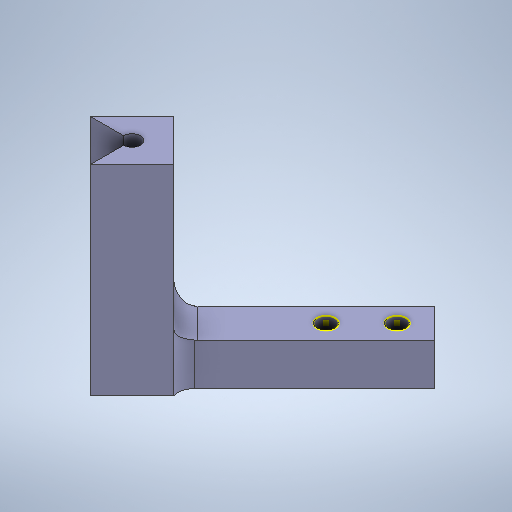
# Autodesk Inventor part: ALUMFINGER
Saved by Autodesk Inventor 2025.2 (Build 292293000, 293)
## iProperties
Created: 2025-02-25
Part Number: ALUMFINGER
Material: Generic
Document SubType Name: Modeling
Designer: m_kni
Density: 1 g/cm^3
Appearance: Default
Author: m_kni
## iProperties of the stored document ALUMFINGER_3DPrint.ipt
Created: 2025-03-03
Part Number: ALUMFINGER_3DPrint
Material: Generic
Document SubType Name: Modeling
Designer: m_kni
Density: 1 g/cm^3
Appearance: Default
Author: m_kni
Autodesk Inventor part; units mm, degrees
ref_plane "YZ Plane" through (0, 0, 0) normal (1, 0, 0) x (0, 1, 0)
ref_plane "XZ Plane" through (0, 0, 0) normal (0, 1, 0) x (-1, 0, 0)
ref_plane "XY Plane" through (0, 0, 0) normal (0, 0, 1) x (1, 0, 0)
sketch "Sketch1" plane through (0, 0, 0) normal (0, 1, 0) x (-1, 0, 0)
  arc A0 (-0.1589, 2.5271) -> (-1.6479, 1.8018) centre (0.1482, 0.0058) ccw
  arc A1 (-0.1589, 2.5271) -> (-1.6479, 1.8018) centre (0.1482, 0.0058) ccw
  arc A2 (1.9442, -1.7903) -> (2.6695, -0.3013) centre (0.1482, 0.0058) ccw
  arc A3 (1.9442, -1.7903) -> (2.6695, -0.3013) centre (0.1482, 0.0058) ccw
  arc A4 (0.1482, 2.5458) -> (-1.6479, 1.8018) centre (0.1482, 0.0058) ccw
  line L0 (0.1482, 5.0058) -> (0.1482, 2.5458)
  line L1 (0.1482, 0.0058) -> (2.6882, 0.0058)
  line L2 (-1.6479, 1.8018) -> (-4.1479, -0.6982)
  arc A5 (1.9442, -1.7903) -> (2.6882, 0.0058) centre (0.1482, 0.0058) ccw
  line L3 (-4.1479, -0.6982) -> (-4.8518, 0.0058)
  arc A6 (0.1482, 2.5458) -> (-1.6479, 1.8018) centre (0.1482, 0.0058) ccw
  arc A7 (0.1482, 2.5458) -> (-1.6479, 1.8018) centre (0.1482, 0.0058) ccw
  arc A8 (-0.1589, 2.5271) -> (-1.6479, 1.8018) centre (0.1482, 0.0058) ccw
  arc A9 (-0.1589, 2.5271) -> (-1.6479, 1.8018) centre (0.1482, 0.0058) ccw
  line L4 (-4.8518, 0.0058) -> (0.1482, 5.0058)
  line L5 (-4.8518, 0.0058) -> (0.1482, 5.0058)
  line L6 (0.1482, 5.0058) -> (0.1482, 2.5458)
  arc A10 (0.1482, 2.5458) -> (-1.6479, 1.8018) centre (0.1482, 0.0058) ccw
  line L7 (-1.6479, 1.8018) -> (-4.1479, -0.6982)
  line L8 (-4.1479, -0.6982) -> (-4.8518, 0.0058)
  arc A11 (1.9442, -1.7903) -> (2.6882, 0.0058) centre (0.1482, 0.0058) ccw
  arc A12 (1.9442, -1.7903) -> (2.6695, -0.3013) centre (0.1482, 0.0058) ccw
  arc A13 (1.9442, -1.7903) -> (2.6695, -0.3013) centre (0.1482, 0.0058) ccw
  arc A14 (1.9442, -1.7903) -> (2.6882, 0.0058) centre (0.1482, 0.0058) ccw
  line L9 (-4.1479, -0.6982) -> (-0.5558, -4.2903)
  line L10 (0.1482, 1.0058) -> (0.1482, 0.0058)
  line L11 (0.1482, 1.0058) -> (0.1482, 0.0058)
  line L12 (0.1482, 2.5458) -> (0.1482, 0.0058)
  line L13 (0.1482, 5.0058) -> (0.1482, 2.5458)
  line L14 (0.1482, 5.0058) -> (0.1482, 1.0058)
  line L15 (0.1482, 0.0058) -> (1.1482, 0.0058)
  line L16 (1.1482, 0.0058) -> (5.1482, 0.0058)
  line L17 (2.6882, 0.0058) -> (5.1482, 0.0058)
  line L18 (0.1482, 0.0058) -> (2.6882, 0.0058)
  line L19 (5.1482, 0.0058) -> (0.1482, -4.9942)
  line L20 (0.1482, -4.9942) -> (5.1482, 0.0058)
  line L21 (-4.1479, -0.6982) -> (-4.8518, 0.0058)
  line L22 (-4.1479, -0.6982) -> (-0.5558, -4.2903)
  line L23 (0.1482, -4.9942) -> (-0.5558, -4.2903)
  line L24 (-4.8518, 0.0058) -> (0.1482, -4.9942)
  line L25 (-4.8518, 0.0058) -> (0.1482, -4.9942)
  line L26 (0.1482, 5.0058) -> (-4.8518, 0.0058)
  line L27 (-4.8518, 0.0058) -> (0.1482, 5.0058)
  line L28 (0.1482, 5.0058) -> (-4.8518, 0.0058)
  line L29 (0.1482, -4.9942) -> (-0.5558, -4.2903)
  arc A15 (1.9442, -1.7903) -> (2.6882, 0.0058) centre (0.1482, 0.0058) ccw
  line L30 (-0.5558, -4.2903) -> (1.9442, -1.7903)
  line L31 (2.6882, 0.0058) -> (5.1482, 0.0058)
  line L32 (5.1482, 0.0058) -> (0.1482, -4.9942)
  line L33 (0.1482, -4.9942) -> (-0.5558, -4.2903)
  line L34 (-0.5558, -4.2903) -> (1.9442, -1.7903)
  arc A16 (1.9442, -1.7903) -> (2.6882, 0.0058) centre (0.1482, 0.0058) ccw
  line L35 (2.6882, 0.0058) -> (5.1482, 0.0058)
  line L36 (5.1482, 0.0058) -> (0.1482, -4.9942)
  arc A17 (0.1482, 2.5458) -> (-1.6479, 1.8018) centre (0.1482, 0.0058) ccw
  circle A18 centre (-2.355, -2.4974) radius 1.5
  circle A19 centre (-2.355, -2.4974) radius 1.5
  circle A20 centre (-2.355, -2.4974) radius 1.5
  circle A21 centre (-2.355, -2.4974) radius 1.5
  circle A22 centre (-2.355, -2.4974) radius 1.5
  line L37 (0.1482, 5.0058) -> (0.1482, 1.0058)
  arc A23 (0.1482, 1.0058) -> (1.1482, 0.0058) centre (0.1482, 0.0058) ccw
  line L38 (0.1482, -4.9942) -> (5.1482, 0.0058)
  line L39 (1.1482, 0.0058) -> (5.1482, 0.0058)
  line L40 (0.1482, 0.0058) -> (1.1482, 0.0058)
  arc A24 (0.1482, 1.0058) -> (1.1482, 0.0058) centre (0.1482, 0.0058) ccw
  line L41 (0.1482, 0.0058) -> (1.1482, 0.0058)
  line L42 (0.1482, 1.0058) -> (0.1482, 0.0058)
  arc A25 (0.1482, 1.0058) -> (1.1482, 0.0058) centre (0.1482, 0.0058) ccw
  arc A26 (0.1482, 1.0058) -> (1.1482, 0.0058) centre (0.1482, 0.0058) ccw
  arc A27 (0.1482, 1.0058) -> (1.1482, 0.0058) centre (0.1482, 0.0058) ccw
  line L43 (0.1482, 5.0058) -> (-4.8518, 0.0058)
  line L44 (-4.8518, 0.0058) -> (0.1482, -4.9942)
  line L45 (0.1482, -4.9942) -> (5.1482, 0.0058)
  line L46 (1.1482, 0.0058) -> (5.1482, 0.0058)
  arc A28 (0.1482, 1.0058) -> (1.1482, 0.0058) centre (0.1482, 0.0058) ccw
  line L47 (0.1482, 5.0058) -> (0.1482, 1.0058)
  line L48 (0.1482, 2.5458) -> (0.1482, 0.0058)
  arc A29 (-1.6479, 1.8018) -> (1.9442, -1.7903) centre (0.1482, 0.0058) ccw
  circle A30 centre (0.1482, 0.0058) radius 2.54
  line L49 (0.1482, -3.5863) -> (-3.4439, 0.0058)
  line L50 (-1.6479, -1.7903) -> (-2.355, -2.4974)
  circle A31 centre (-2.355, -2.4974) radius 2.54
  point P0 (0, 0)
  point P1 (1.1482, 0.0058)
  constraints: 86 end point, 44 point on circle, 28 centre point, 38 other
extrude "Extrusion1" add sketch "Sketch1" along normal blind 23.9 contours A4 L12 A23 A31 A29 A0 | A0 L2 L3 L4 L0 A4 | A29 A31 L49 L2 | L49 A31 L2 | A31 A29 A18 | A29 A18 L49 A31 | A5 A2 A29 A31 A23 L1 | L16 L19 L23 L30 A2 A5 | A31 L49 A18 L9 | A29 L49 A18 | A18 A29 | A18 L49 L50 L9 | A31 L49 L30 | L9 A18 L49 A31 | A29 A31 L49 A18 | A18 L49 A29 | L49 A18 L9 L50 | L30 L49 A31 A29
sketch "Sketch2" plane through (0, 0, 0) normal (0, -1, 0) x (1, 0, 0)
  line L0 (4.8518, 0.0058) -> (-0.1482, -4.9942) projected
  line L1 (2.3518, -2.4942) -> (17.9082, -18.0506)
  circle A0 centre (11.4481, -11.5905) radius 1.075
  circle A1 centre (15.6907, -15.8331) radius 1.075
  line L2 (-0.1482, 1.0058) -> (-0.1482, 5.0058) projected
  line L3 (-0.1482, 5.0058) -> (4.8518, 0.0058)
  line L4 (-0.1482, 5.0058) -> (4.8518, 0.0058) projected
  line L5 (-0.1482, -4.9942) -> (-5.1482, 0.0058) projected
  line L6 (-5.1482, 0.0058) -> (-0.1482, -4.9942)
  line L7 (2.3518, -2.4942) -> (4.1196, -0.7265)
  line L8 (4.1196, -0.7265) -> (0.5841, -4.262)
  line L9 (0.5841, -4.262) -> (16.0443, -19.7222)
  line L10 (4.1196, -0.7265) -> (19.5798, -16.1867)
  line L11 (17.9082, -18.0506) -> (17.812, -18.1468)
  line L12 (17.812, -18.1468) -> (16.1404, -19.8184)
  line L13 (16.1404, -19.8184) -> (16.0443, -19.7222)
  line L14 (17.9082, -18.0506) -> (19.676, -16.2828)
  line L15 (19.676, -16.2828) -> (19.5798, -16.1867)
  point P0 (0, 0)
  dimension "d2" = 22
  dimension "d5" = 2.15
  dimension "d6" = 2.15
  dimension "d7" = 2.5
  dimension "d8" = 5
  constraints: 24 end point, 8 point on line, 3 perpendicular, 2 centre point, 2 collinear, 1 midpoint
  measures "d2" distance of L1.start L1.end
  measures "d5" diameter of A0
  measures "d6" diameter of A1
  measures "d7" distance of L1.start L7.end
  measures "d8" distance of L7.end L8.end
extrude "Extrusion2" add sketch "Sketch2" against normal blind 5 contours L10 L15 L14 L1 A1 A0 L0 | L1 A0 A1 L11 L12 L13 L9 L0
fillet "Fillet1" radius 2 2 edges at (4.1196, 2.5, -0.7265) (0.5841, 2.5, -4.262)
fillet "Fillet2" radius 2 1 edges at (2.3518, 5, -2.4942)
sketch "Sketch3" plane through (0, 5, 0) normal (0, 1, 0) x (1, 0, 0)
  circle A0 centre (11.4481, 11.5905) radius 1.075 projected
  circle A1 centre (15.6907, 15.8331) radius 1.075 projected
  point P0 (0, 0)
body "Solid1"
